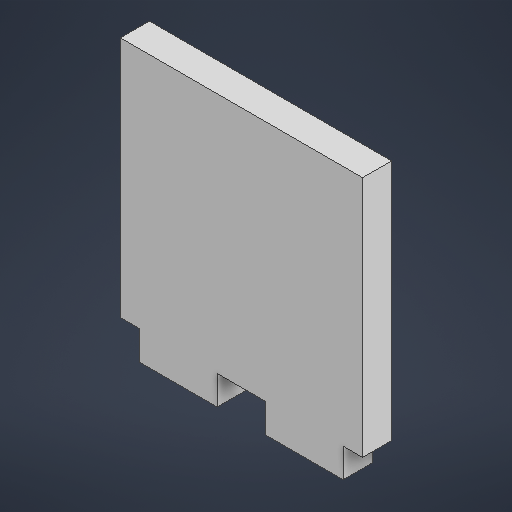
# Autodesk Inventor part: protector hal
Saved by Autodesk Inventor 2026 (Build 300175000, 175)
## iProperties
Created: 2026-05-15
Part Number: protector hal
Material: Generic
Document SubType Name: Modeling
Designer: juana
Density: 1 g/cm^3
Appearance: Default
Author: juana
Autodesk Inventor part; units mm, degrees
ref_plane "YZ Plane" through (0, 0, 0) normal (1, 0, 0) x (0, 1, 0)
ref_plane "XZ Plane" through (0, 0, 0) normal (0, 1, 0) x (-1, 0, 0)
ref_plane "XY Plane" through (0, 0, 0) normal (0, 0, 1) x (1, 0, 0)
sketch "Sketch1" plane through (0, 0, 0) normal (0, 0, 1) x (1, 0, 0)
  line L0 (0, 0) -> (25, 0)
  line L1 (25, 0) -> (25, 25)
  line L2 (25, 25) -> (0, 25)
  line L3 (0, 25) -> (0, 0)
  line L4 (2, 0) -> (10, 0)
  line L5 (10, 0) -> (10, -3)
  line L6 (10, -3) -> (2, -3)
  line L7 (2, -3) -> (2, 0)
  line L8 (12.5, 0) -> (12.5, 25) construction
  line L9 (0, 12.5) -> (25, 12.5) construction
  line L10 (15, 0) -> (15, -3)
  line L11 (15, -3) -> (23, -3)
  line L12 (23, -3) -> (23, 0)
  point P0 (23, 0)
  point P1 (15, 0)
  point P2 (10, 0)
  dimension "d0" = 25
  dimension "d1" = 25
  dimension "d5" = 3
  dimension "d6" = 2
  dimension "d7" = 8
  constraints: 26 end point, 4 midpoint, 4 parallel, 4 symmetric about line, 2 horizontal, 2 perpendicular, 1 point on line
  measures "d0" distance of L1.end L2.end
  measures "d1" distance of L0.end L1.end
  measures "d5" distance of L4.end L5.end
  measures "d6" distance between parallel lines of L3 L7
  measures "d7" distance of L5.end L6.end
extrude "Extrusion1" add sketch "Sketch1" along normal blind 3
body "Solid1"
